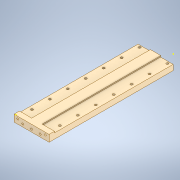
# Autodesk Inventor part: 5212_Bias_TxRx_Relative_Dovetail_Male_MPSv2_v3
Saved by Autodesk Inventor 2021 (Build 250183000, 183)
## iProperties
Created: 2020-11-13
Part Number: 5212_Bias_TxRx_Relative_Dovetail_Male_MPSv2_v3
Material: Polyethylene, High Density
Document SubType Name: Modeling
Designer: Admin
Density: 0.952 g/cm^3
Appearance: Smooth - Off-White
Author: Admin
Autodesk Inventor part; units mm, degrees
ref_plane "YZ Plane" through (0, 0, 0) normal (1, 0, 0) x (0, 1, 0)
ref_plane "XZ Plane" through (0, 0, 0) normal (0, 1, 0) x (-1, 0, 0)
ref_plane "XY Plane" through (0, 0, 0) normal (0, 0, 1) x (1, 0, 0)
sketch "Sketch1" plane through (0, 0, 0) normal (0, 0, 1) x (1, 0, 0)
  line L0 (38.0718, -21.4) -> (37, -25.4)
  line L1 (37, -25.4) -> (38.0718, -21.4)
  line L2 (8.9282, -21.4) -> (38.0718, -21.4)
  line L3 (38.0718, -21.4) -> (8.9282, -21.4)
  line L4 (10, -25.4) -> (8.9282, -21.4)
  line L5 (8.9282, -21.4) -> (10, -25.4)
  line L6 (10, -25.4) -> (0, -25.4)
  line L7 (10, -25.4) -> (0, -25.4)
  line L8 (47, -25.4) -> (37, -25.4)
  line L9 (37, -25.4) -> (47, -25.4)
  line L10 (38.0718, -21.4) -> (37, -25.4)
  line L11 (37, -25.4) -> (38.0718, -21.4)
  line L12 (8.9282, -21.4) -> (38.0718, -21.4)
  line L13 (38.0718, -21.4) -> (8.9282, -21.4)
  line L14 (10, -25.4) -> (8.9282, -21.4)
  line L15 (8.9282, -21.4) -> (10, -25.4)
  line L16 (10, -25.4) -> (0, -25.4)
  line L17 (10, -25.4) -> (0, -25.4)
  line L18 (47, -25.4) -> (37, -25.4)
  line L19 (37, -25.4) -> (47, -25.4)
  line L20 (0, -38.1) -> (47, -38.1)
  line L21 (47, -25.4) -> (72.4, -25.4)
  line L22 (72.4, -25.4) -> (72.4, -38.1)
  line L23 (72.4, -38.1) -> (47, -38.1)
  line L24 (0, -25.4) -> (-25.4, -25.4)
  line L25 (-25.4, -25.4) -> (-25.4, -38.1)
  line L26 (-25.4, -38.1) -> (0, -38.1)
  point P0 (0, 0)
  point P1 (0, 0)
  point P2 (0, 0)
  dimension "d52" = 4
  dimension "d53" = 27
  dimension "d54" = 29.1436
  constraints: 54 end point, 12 equal length, 2 horizontal, 2 perpendicular
  measures "d52" vertical distance of L0.start L0.end
  measures "d53" distance of L4.start L0.end
  measures "d54" distance of L2.start L0.start
extrude "Extrusion1" add sketch "Sketch1" along normal blind 331
sketch "Sketch4" plane through (0, 0, 0) normal (0, 0, -1) x (-1, 0, 0)
  line L0 (-38.0718, -21.4) -> (-8.9282, -21.4) projected
  line L1 (-8.9282, -21.4) -> (-8.9282, -38.1)
  line L2 (25.4, -38.1) -> (-72.4, -38.1) projected
  line L3 (25.4, -38.1) -> (25.4, -40.45)
  line L4 (25.4, -40.45) -> (-72.4, -40.45)
  line L5 (-72.4, -40.45) -> (-72.4, -38.1)
  line L6 (-72.4, -38.1) -> (25.4, -38.1)
  line L7 (25.4, -38.1) -> (25.4, -40.45)
  point P0 (0, 0)
  dimension "d26" = 2.35
  constraints: 12 end point, 2 parallel, 2 vertical, 1 horizontal, 1 perpendicular, 1 point on line
  measures "d26" distance of L2.start L3.end
extrude "Extrusion4" add sketch "Sketch4" against normal blind 331
sketch "Sketch3" plane through (37, -25.4, 331) normal (0, 1, 0) x (1, 0, 0)
  line L0 (35.4, 0) -> (0, 0) projected
  line L1 (-28.0718, 0) -> (-27, 0) projected
  line L2 (0, 0) -> (-27, 0)
  line L3 (-27, 0) -> (-13.5, 0)
  line L4 (-13.5, 0) -> (-13.5, 11.6369)
  line L5 (-13.5, 0) -> (-1.8631, 0) construction
  line L6 (35.4, 0) -> (25.4, 0)
  line L7 (25.4, 0) -> (25.4, 25)
  line L8 (25.4, 25) -> (25.4, 75)
  line L9 (25.4, 75) -> (25.4, 125)
  line L10 (25.4, 125) -> (25.4, 175)
  line L11 (25.4, 175) -> (25.4, 225)
  line L12 (25.4, 225) -> (25.4, 275)
  line L13 (25.4, 275) -> (25.4, 325)
  circle A0 centre (25.4, 325) radius 3.175
  circle A1 centre (25.4, 275) radius 3.175
  circle A2 centre (25.4, 225) radius 3.175
  circle A3 centre (25.4, 175) radius 3.175
  circle A4 centre (25.4, 125) radius 3.175
  circle A5 centre (25.4, 75) radius 3.175
  circle A6 centre (25.4, 25) radius 3.175
  circle A7 centre (-52.4, 325) radius 3.175
  circle A8 centre (-52.4, 275) radius 3.175
  circle A9 centre (-52.4, 225) radius 3.175
  circle A10 centre (-52.4, 175) radius 3.175
  circle A11 centre (-52.4, 125) radius 3.175
  circle A12 centre (-52.4, 75) radius 3.175
  circle A13 centre (-52.4, 25) radius 3.175
  point P0 (-37, 331)
  dimension "d8" = 90
  dimension "d9" = 10
  dimension "d10" = 25
  dimension "d11" = 50
  dimension "d12" = 50
  dimension "d13" = 50
  dimension "d14" = 50
  dimension "d15" = 50
  dimension "d16" = 50
  dimension "d17" = 6.35
  dimension "d18" = 6.35
  dimension "d19" = 6.35
  dimension "d20" = 6.35
  dimension "d21" = 6.35
  dimension "d22" = 6.35
  dimension "d23" = 6.35
  constraints: 24 end point, 14 centre point, 7 coincident, 7 point on line, 7 symmetric about line, 2 horizontal, 2 perpendicular, 1 midpoint, 7 other
  measures "d8" angle of L5 L4
  measures "d9" distance of L0.start L6.end
  measures "d10" distance of L6.end L7.end
  measures "d11" distance of L7.end L8.end
  measures "d12" distance of L8.end L9.end
  measures "d13" distance of L9.end L10.end
  measures "d14" distance of L10.end L11.end
  measures "d15" distance of L11.end L12.end
  measures "d16" distance of L12.end L13.end
  measures "d17" diameter of A0
  measures "d18" diameter of A1
  measures "d19" diameter of A2
  measures "d20" diameter of A3
  measures "d21" diameter of A4
  measures "d22" diameter of A5
  measures "d23" diameter of A6
extrude "Extrusion3" cut sketch "Sketch3" against normal blind 300
sketch "Sketch5" plane through (0, 0, 331) normal (0, 0, 1) x (1, 0, 0)
  line L0 (37, -25.4) -> (38.0718, -21.4) projected
  line L1 (38.0718, -21.4) -> (72.4488, -21.4)
  line L2 (72.4488, -40.7637) -> (72.4488, -13.0005)
  line L3 (-25.4, -25.4) -> (-25.4, -40.45) projected
  line L4 (72.4488, -21.4) -> (-25.4, -21.4)
  line L5 (-25.4, -21.4) -> (-25.4, -40.45)
  line L6 (-25.4, -40.45) -> (72.4488, -40.45)
  line L7 (72.4488, -40.45) -> (72.4488, -21.4)
  point P0 (0, 0)
  constraints: 12 end point, 2 horizontal, 2 parallel, 1 perpendicular, 1 vertical
extrude "Extrusion5" add sketch "Sketch5" along normal blind 35
sketch "Sketch6" plane through (0, 0, 366) normal (0, 0, 1) x (1, 0, 0)
  point P0 (0, 0)
sketch "Sketch7" plane through (72.4, -40.45, 0) normal (1, 0, 0) x (0, 0, -1)
  point P0 (0, 40.45)
sketch "Sketch8" plane through (0, 0, 366) normal (0, 0, 1) x (1, 0, 0)
  line L0 (-25.4, -21.4) -> (-25.4, -40.45) projected
  line L1 (-25.4, -21.4) -> (-25.4, -25.4)
  line L2 (72.4, -40.45) -> (72.4488, -40.45) projected
  line L3 (-25.4, -25.4) -> (72.4488, -40.45)
  line L4 (72.4, -40.45) -> (72.4, -25.4) projected
  line L5 (72.4488, -40.45) -> (72.4, -25.4)
  line L6 (72.4, -25.4) -> (-25.4, -40.45)
  line L7 (23.5, -32.925) -> (-0.95, -32.925)
  line L8 (-0.95, -32.925) -> (47.95, -32.925)
  circle A0 centre (-0.95, -32.925) radius 2.5
  circle A1 centre (23.5, -33.0837) radius 2.5
  circle A2 centre (47.95, -32.925) radius 2.5
  point P0 (0, 0)
  point P1 (-25.4, -38.1)
  dimension "d31" = 4
  dimension "d32" = 24.45
  dimension "d33" = 48.9
  dimension "d34" = 5
  dimension "d35" = 5
  dimension "d36" = 5
  constraints: 12 end point, 3 centre point, 3 point on line, 2 coincident, 1 horizontal, 1 midpoint
  measures "d31" distance of L0.start L1.end
  measures "d32" distance of L7.start L7.end
  measures "d33" distance of L7.end L8.end
  measures "d34" diameter of A0
  measures "d35" diameter of A1
  measures "d36" diameter of A2
extrude "Extrusion6" cut sketch "Sketch8" against normal blind 30 contours A0 | A1 L6 L3 | L3 L7 A1 | A1 L7 L6 | L6 L3 A1 | A1 L8 L6 | A2 | L3 L8 A1
sketch "Sketch9" plane through (0, 0, 366) normal (0, 0, 1) x (1, 0, 0)
  circle A0 centre (-0.95, -32.925) radius 2.5 projected
  line L0 (-0.95, -32.925) -> (13.1454, -27.7947)
  line L1 (-0.95, -32.925) -> (14.05, -32.925) construction
  line L2 (-0.95, -32.925) -> (-15.0454, -27.7947)
  line L3 (-0.95, -32.925) -> (14.05, -32.925) construction
  circle A1 centre (47.95, -32.925) radius 2.5 projected
  line L4 (47.95, -32.925) -> (62.0454, -27.7947)
  line L5 (47.95, -32.925) -> (62.95, -32.925) construction
  circle A2 centre (-15.0454, -27.7947) radius 2.5
  circle A3 centre (62.0454, -27.7947) radius 2.5
  point P0 (0, 0)
  dimension "d39" = 15
  dimension "d40" = 20
  dimension "d41" = 15
  dimension "d42" = 160
  dimension "d43" = 15
  dimension "d44" = 20
  dimension "d45" = 5
  dimension "d46" = 5
  constraints: 12 end point, 3 equal length, 3 horizontal, 2 centre point, 2 coincident
  measures "d39" distance of L0.start L0.end
  measures "d40" angle of L1 L0
  measures "d41" distance of L0.start L2.end
  measures "d42" angle of L3 L2
  measures "d43" distance of L4.start L4.end
  measures "d44" angle of L5 L4
  measures "d45" diameter of A2
  measures "d46" diameter of A3
extrude "Extrusion7" cut sketch "Sketch9" against normal blind 30 contours A2 | A3
sketch "Sketch10" plane through (8.9282, -21.4, 0) normal (0, 1, 0) x (1, 0, 0)
  line L0 (-34.3282, -331) -> (-34.3282, -366) projected
  line L1 (63.5206, -331) -> (63.5206, -366) projected
  line L2 (-34.3282, -366) -> (63.5206, -366)
  line L3 (63.5206, -366) -> (63.5206, -331)
  line L4 (63.5206, -331) -> (-34.3282, -331)
  line L5 (-34.3282, -331) -> (-34.3282, -366)
  line L6 (63.4718, 0) -> (63.4718, -331) projected
  line L7 (63.4718, -331) -> (-34.3282, -331)
  line L8 (-34.3282, -331) -> (-34.3282, -346)
  line L9 (-34.3282, -346) -> (63.4718, -346)
  line L10 (63.4718, -346) -> (63.4718, -331)
  point P0 (-8.9282, 0)
  point P1 (-34.3282, -346)
  dimension "d49" = 15
  constraints: 16 end point, 4 parallel, 2 horizontal, 2 perpendicular, 1 point on line
  measures "d49" distance of L8.end L7.end
extrude "Extrusion8" cut sketch "Sketch10" against normal blind 30 contours L9 L10 L4 L1 L2 L0
body "Solid1"
